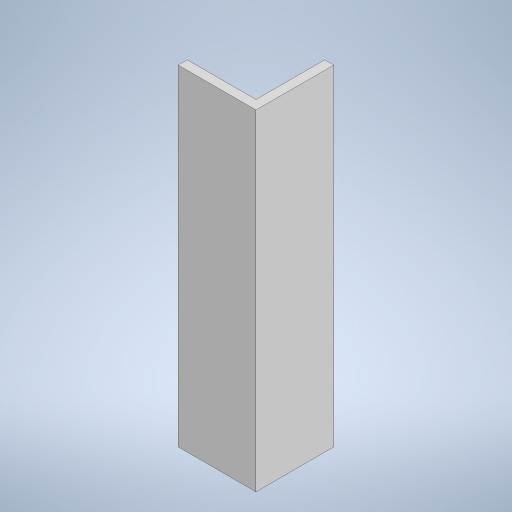
# Autodesk Inventor part: corners
Saved by Autodesk Inventor 2023 (Build 270158000, 158)
## iProperties
Created: 2022-09-23
Part Number: corners
Material: Generic
Document SubType Name: Modeling
Designer: Desmond
Density: 1 g/cm^3
Appearance: Default
Author: Desmond
Autodesk Inventor part; units mm, degrees
ref_plane "YZ Plane" through (0, 0, 0) normal (1, 0, 0) x (0, 1, 0)
ref_plane "XZ Plane" through (0, 0, 0) normal (0, 1, 0) x (-1, 0, 0)
ref_plane "XY Plane" through (0, 0, 0) normal (0, 0, 1) x (1, 0, 0)
sketch "Sketch1" plane through (0, 0, 0) normal (0, 1, 0) x (-1, 0, 0)
  line L0 (0, 0) -> (12, 0)
  line L1 (12, 0) -> (12, -1.4)
  line L2 (12, -1.4) -> (0, -1.4)
  line L3 (0, -1.4) -> (0, 0)
  line L4 (0, -1.4) -> (1.4, -1.4)
  line L5 (1.4, -1.4) -> (1.4, -12)
  line L6 (1.4, -12) -> (0, -12)
  line L7 (0, -12) -> (0, -1.4)
  dimension "d0" = 12
  dimension "d1" = 1.4
  dimension "d2" = 1.4
  dimension "d3" = 10.6
  constraints: 16 end point, 4 parallel, 2 horizontal, 2 perpendicular
  measures "d0" distance of L1.end L2.end
  measures "d1" distance of L0.end L1.end
  measures "d2" distance of L5.end L6.end
  measures "d3" distance of L4.end L5.end
extrude "Extrusion1" add sketch "Sketch1" along normal blind 51
body "Solid1"
